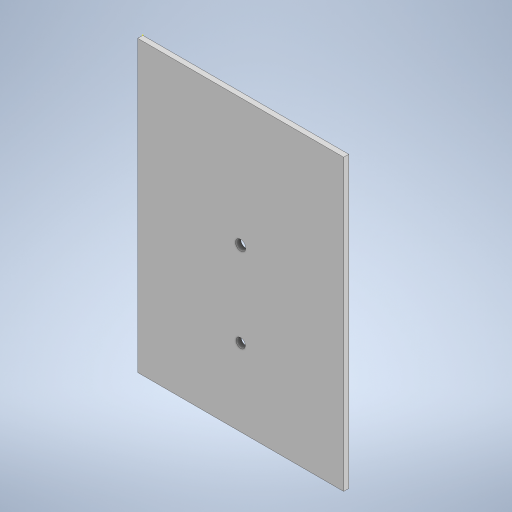
# Autodesk Inventor part: platform-mount
Saved by Autodesk Inventor 2024 (Build 280153000, 153)
## iProperties
Created: 2024-04-14
Part Number: platform-mount
Material: Generisch
Document SubType Name: Modeling
Designer: anash
Density: 1 g/cm^3
Appearance: Vorgabe
Author: anash
Autodesk Inventor part; units mm, degrees
ref_plane "YZ Plane" through (0, 0, 0) normal (1, 0, 0) x (0, 1, 0)
ref_plane "XZ Plane" through (0, 0, 0) normal (0, 1, 0) x (-1, 0, 0)
ref_plane "XY Plane" through (0, 0, 0) normal (0, 0, 1) x (1, 0, 0)
sketch "Skizze1" plane through (0, 0, 0) normal (0, 1, 0) x (-1, 0, 0)
  line L0 (0, 0) -> (-121, 0)
  line L1 (-121, 0) -> (-121, -170)
  line L2 (-121, -170) -> (0, -170)
  line L3 (0, -170) -> (0, 0)
  circle A0 centre (-60.5, -75) radius 3
  circle A1 centre (-60.5, -124.75) radius 2.75
  dimension "d0" = 121
  dimension "d1" = 170
  dimension "d2" = 75
  dimension "d3" = 6
  dimension "d4" = 60.5
  dimension "d5" = 49.75
  dimension "d6" = 60.5
  dimension "d7" = 5.5
  constraints: 8 end point, 2 centre point, 2 parallel, 1 horizontal, 1 perpendicular
  measures "d0" distance of L2.end L1.end
  measures "d1" distance of L1.end L0.end
  measures "d2" distance from line of L0 A0.centre
  measures "d3" diameter of A0
  measures "d4" distance from line of L3 A0.centre
  measures "d5" distance of A1.centre A0.centre
  measures "d6" distance from line of L3 A1.centre
  measures "d7" diameter of A1
extrude "Extrusion1" add sketch "Skizze1" along normal blind 3
sketch "Skizze6" plane through (0, 3, 0) normal (0, 1, 0) x (1, 0, 0)
  line L0 (27.5, 15) -> (93.5, 15)
  line L1 (93.5, 15) -> (93.5, 65)
  line L2 (93.5, 65) -> (27.5, 65)
  line L3 (27.5, 65) -> (27.5, 15)
  line L4 (0, 170) -> (0, 0) projected
  line L5 (0, 0) -> (121, 0) projected
  dimension "d72" = 66
  dimension "d73" = 50
  dimension "d74" = 27.5
  dimension "d75" = 15
  constraints: 8 end point, 2 parallel, 1 horizontal, 1 perpendicular
  measures "d72" distance between parallel lines of L1 L3
  measures "d73" distance between parallel lines of L2 L0
  measures "d74" distance between parallel lines of L4 L3
  measures "d75" distance between parallel lines of L0 L5
extrude "Extrusion6" add sketch "Skizze6" along normal blind 15
sketch "Skizze7" plane through (27.5, 3, -15) normal (0, 0, 1) x (1, 0, 0)
  line L0 (66, 15) -> (0, 15) projected
  line L1 (0, 0) -> (66, 0) projected
  line L2 (15, 15) -> (51, 15)
  line L3 (51, 15) -> (51, 0)
  line L4 (51, 0) -> (15, 0)
  line L5 (15, 0) -> (15, 15)
  line L6 (0, 0) -> (0, 15) projected
  line L7 (0, 0) -> (21.2132, 0) construction
  line L8 (66, 0) -> (87.2132, 0) construction
  line L9 (66, 0) -> (66, 15) projected
  line L10 (93.5, 0) -> (-27.5, 0) projected
  line L11 (5, 0) -> (15, 10)
  line L12 (5, 0) -> (19.1421, 0) construction
  line L13 (51, 10) -> (61, 0)
  line L14 (51, 10) -> (65.1421, 10) construction
  line L15 (15, 15) -> (51, 15)
  line L16 (51, 15) -> (51, 10)
  line L17 (51, 10) -> (15, 10)
  line L18 (15, 10) -> (15, 15)
  point P0 (-27.5, -3)
  dimension "d78" = 36
  dimension "d79" = 15
  dimension "d85" = 45
  dimension "d86" = 45
  constraints: 28 end point, 6 horizontal, 4 parallel, 4 point on line, 2 equal length, 2 perpendicular, 3 other
  measures "d78" distance between parallel lines of L3 L5
  measures "d79" distance between parallel lines of L5 L6
  measures "d85" angle of L12 L11
  measures "d86" angle of L13 L14
extrude "Extrusion7" cut sketch "Skizze7" against normal blind 40 contours L3 L17 L5 L0 | L13 L1 L3 | L3 L1 L5 L17 | L5 L1 L11
sketch "Skizze8" plane through (0, 3, 0) normal (0, 1, 0) x (1, 0, 0)
  point P0 (0, 0)
